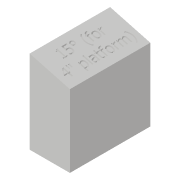
# Autodesk Inventor part: 15DegreeStand
Saved by Autodesk Inventor 2018 (Build 220112000, 112)
## iProperties
Created: 2018-12-13
Part Number: 15DegreeStand
Material: Generic
Document SubType Name: Modeling
Designer: ball
Density: 1 g/cm^3
Appearance: Default
Author: ball
Autodesk Inventor part; units mm, degrees
ref_plane "YZ Plane" through (0, 0, 0) normal (1, 0, 0) x (0, 1, 0)
ref_plane "XZ Plane" through (0, 0, 0) normal (0, 1, 0) x (-1, 0, 0)
ref_plane "XY Plane" through (0, 0, 0) normal (0, 0, 1) x (1, 0, 0)
sketch "Sketch1" plane through (0, 0, 0) normal (0, 1, 0) x (-1, 0, 0)
  line L0 (0, 0) -> (12.7, 0)
  line L1 (12.7, 0) -> (12.7, -25.4)
  line L2 (12.7, -25.4) -> (0, -25.4)
  line L3 (0, -25.4) -> (0, 0)
  dimension "d0" = 12.7
  dimension "d1" = 25.4
  constraints: 8 end point, 2 parallel, 1 horizontal, 1 perpendicular
  measures "d0" distance of L1.end L2.end
  measures "d1" distance of L0.end L1.end
extrude "Extrusion1" add sketch "Sketch1" along normal blind 26.289
sketch "Sketch2" plane through (-12.7, 0, 0) normal (0, 0, 1) x (1, 0, 0)
  line L0 (0, 0) -> (0, 26.289) projected
  line L1 (0, 26.289) -> (12.7, 26.289) projected
  line L2 (0, 26.289) -> (12.7, 26.289)
  line L3 (0, 26.289) -> (12.7, 22.886)
  line L4 (0, 26.289) -> (13.148, 26.289) construction
  line L5 (12.7, 0) -> (12.7, 26.289) projected
  line L6 (12.7, 22.886) -> (12.7, 26.289)
  dimension "d4" = 15
  constraints: 8 end point, 1 collinear, 1 equal length, 1 horizontal, 1 perpendicular
  measures "d4" angle of L3 L4
extrude "Extrusion2" cut sketch "Sketch2" against normal blind 26.289
sketch "Sketch3" plane through (-12.7, 26.289, 0) normal (0.258819, 0.9659258, 0) x (0.9659258, -0.258819, 0)
  line L0 (2.3231, -6.9377) -> (2.3231, 32.6962) construction
  line L1 (2.3231, 32.6962) -> (11.3899, 32.6962) construction
  line L2 (11.3899, 32.6962) -> (11.3899, -6.9377) construction
  line L3 (11.3899, -6.9377) -> (2.3231, -6.9377) construction
  line L4 (5.5267, 6.8821) -> (5.5267, 5.3951)
  line L5 (5.5267, 5.3951) -> (5.2155, 5.3951)
  line L6 (5.2155, 5.3951) -> (5.2155, 5.9484)
  line L7 (5.2155, 5.9484) -> (3.1727, 5.9484)
  line L8 (3.1727, 5.9484) -> (3.1727, 5.3951)
  line L9 (3.1727, 5.3951) -> (2.8936, 5.3951)
  spline S0 degree 2 poles (2.8936, 5.3951) (2.8936, 5.7088) (2.7158, 6.0052) (2.4688, 6.025) knots 0 0 0 1 2 2 2
  line L10 (2.4688, 6.025) -> (2.4688, 6.3411)
  line L11 (2.4688, 6.3411) -> (5.2155, 6.3411)
  line L12 (5.2155, 6.3411) -> (5.2155, 6.8821)
  line L13 (5.2155, 6.8821) -> (5.5267, 6.8821)
  spline S1 degree 2 poles (4.5584, 9.2903) (4.7783, 9.2903) (5.1537, 9.1495) (5.292, 9.0211) knots 0 0 0 1 2 2 2
  spline S2 degree 2 poles (5.292, 9.0211) (5.4303, 8.8927) (5.5909, 8.5098) (5.5909, 8.2727) knots 0 0 0 1 2 2 2
  spline S3 degree 2 poles (5.5909, 8.2727) (5.5909, 8.0553) (5.4946, 7.6305) (5.418, 7.4749) knots 0 0 0 1 2 2 2
  line L14 (5.418, 7.4749) -> (4.9857, 7.4749)
  line L15 (4.9857, 7.4749) -> (4.9857, 7.5045)
  spline S4 degree 2 poles (4.9857, 7.5045) (5.0203, 7.5514) (5.1092, 7.7268) (5.1488, 7.833) knots 0 0 0 1 2 2 2
  spline S5 degree 2 poles (5.1488, 7.833) (5.1907, 7.9541) (5.2377, 8.1541) (5.2377, 8.2801) knots 0 0 0 1 2 2 2
  spline S6 degree 2 poles (5.2377, 8.2801) (5.2377, 8.4036) (5.1488, 8.6358) (5.0524, 8.7198) knots 0 0 0 1 2 2 2
  spline S7 degree 2 poles (5.0524, 8.7198) (4.961, 8.7963) (4.719, 8.8754) (4.556, 8.8754) knots 0 0 0 1 2 2 2
  spline S8 degree 2 poles (4.556, 8.8754) (4.3929, 8.8754) (4.1855, 8.7865) (4.1163, 8.7025) knots 0 0 0 1 2 2 2
  spline S9 degree 2 poles (4.1163, 8.7025) (4.0397, 8.616) (3.9755, 8.3591) (3.9755, 8.2035) knots 0 0 0 1 2 2 2
  spline S10 degree 2 poles (3.9755, 8.2035) (3.9755, 8.0356) (4.0274, 7.7021) (4.0496, 7.6008) knots 0 0 0 1 2 2 2
  line L16 (4.0496, 7.6008) -> (2.4787, 7.6008)
  line L17 (2.4787, 7.6008) -> (2.4787, 9.273)
  line L18 (2.4787, 9.273) -> (2.8368, 9.273)
  line L19 (2.8368, 9.273) -> (2.8368, 7.9936)
  line L20 (2.8368, 7.9936) -> (3.6495, 7.9936)
  spline S11 degree 2 poles (3.6495, 7.9936) (3.6396, 8.0677) (3.6322, 8.2109) (3.6322, 8.2702) knots 0 0 0 1 2 2 2
  spline S12 degree 2 poles (3.6322, 8.2702) (3.6322, 8.5049) (3.7087, 8.8284) (3.8224, 8.9766) knots 0 0 0 1 2 2 2
  spline S13 degree 2 poles (3.8224, 8.9766) (3.936, 9.1273) (4.2818, 9.2903) (4.5584, 9.2903) knots 0 0 0 1 2 2 2
  spline S14 degree 2 poles (3.2049, 11.2738) (3.5334, 11.2738) (3.9829, 10.8242) (3.9829, 10.4957) knots 0 0 0 1 2 2 2
  spline S15 degree 2 poles (3.9829, 10.4957) (3.9829, 10.1697) (3.5358, 9.7152) (3.2049, 9.7152) knots 0 0 0 1 2 2 2
  spline S16 degree 2 poles (3.2049, 9.7152) (2.8763, 9.7152) (2.4268, 10.1647) (2.4268, 10.4957) knots 0 0 0 1 2 2 2
  spline S17 degree 2 poles (2.4268, 10.4957) (2.4268, 10.8242) (2.8763, 11.2738) (3.2049, 11.2738) knots 0 0 0 1 2 2 2
  spline S18 degree 2 poles (3.2049, 10.9527) (3.0073, 10.9527) (2.738, 10.6908) (2.738, 10.4957) knots 0 0 0 1 2 2 2
  spline S19 degree 2 poles (2.738, 10.4957) (2.738, 10.2981) (3.0073, 10.0363) (3.2049, 10.0363) knots 0 0 0 1 2 2 2
  spline S20 degree 2 poles (3.2049, 10.0363) (3.4049, 10.0363) (3.6717, 10.303) (3.6717, 10.4957) knots 0 0 0 1 2 2 2
  spline S21 degree 2 poles (3.6717, 10.4957) (3.6717, 10.6908) (3.4, 10.9527) (3.2049, 10.9527) knots 0 0 0 1 2 2 2
  line L21 (6.3689, 14.2427) -> (6.3689, 13.7734)
  spline S22 degree 2 poles (6.3689, 13.7734) (5.9466, 13.4177) (5.0006, 13.0102) (4.3559, 13.0102) knots 0 0 0 1 2 2 2
  spline S23 degree 2 poles (4.3559, 13.0102) (3.726, 13.0102) (2.7652, 13.4128) (2.3428, 13.7734) knots 0 0 0 1 2 2 2
  line L22 (2.3428, 13.7734) -> (2.3428, 14.2427)
  line L23 (2.3428, 14.2427) -> (2.3626, 14.2427)
  spline S24 degree 2 poles (2.3626, 14.2427) (2.5133, 14.0772) (2.9035, 13.7759) (3.1629, 13.6474) knots 0 0 0 1 2 2 2
  spline S25 degree 2 poles (3.1629, 13.6474) (3.4148, 13.5239) (4.02, 13.3708) (4.3559, 13.3708) knots 0 0 0 1 2 2 2
  spline S26 degree 2 poles (4.3559, 13.3708) (4.7066, 13.3708) (5.2871, 13.519) (5.5489, 13.6474) knots 0 0 0 1 2 2 2
  spline S27 degree 2 poles (5.5489, 13.6474) (5.8008, 13.7709) (6.2084, 14.0846) (6.3492, 14.2427) knots 0 0 0 1 2 2 2
  line L24 (6.3492, 14.2427) -> (6.3689, 14.2427)
  line L25 (2.7133, 15.8779) -> (2.7133, 15.8581)
  spline S28 degree 2 poles (2.7133, 15.8581) (2.6936, 15.8062) (2.659, 15.6136) (2.659, 15.537) knots 0 0 0 1 2 2 2
  spline S29 degree 2 poles (2.659, 15.537) (2.659, 15.2949) (2.8763, 15.0875) (3.1629, 15.0875) knots 0 0 0 1 2 2 2
  line L26 (3.1629, 15.0875) -> (3.2394, 15.0875)
  line L27 (3.2394, 15.0875) -> (3.2394, 15.7247)
  line L28 (3.2394, 15.7247) -> (3.5581, 15.7247)
  line L29 (3.5581, 15.7247) -> (3.5581, 15.0998)
  line L30 (3.5581, 15.0998) -> (5.5267, 15.0998)
  line L31 (5.5267, 15.0998) -> (5.5267, 14.7145)
  line L32 (5.5267, 14.7145) -> (3.5581, 14.7145)
  line L33 (3.5581, 14.7145) -> (3.5581, 14.4551)
  line L34 (3.5581, 14.4551) -> (3.2394, 14.4551)
  line L35 (3.2394, 14.4551) -> (3.2394, 14.7145)
  line L36 (3.2394, 14.7145) -> (3.1629, 14.7145)
  spline S30 degree 2 poles (3.1629, 14.7145) (2.7528, 14.7145) (2.3231, 15.1122) (2.3231, 15.4827) knots 0 0 0 1 2 2 2
  spline S31 degree 2 poles (2.3231, 15.4827) (2.3231, 15.5889) (2.3453, 15.7939) (2.3601, 15.8779) knots 0 0 0 1 2 2 2
  line L37 (2.3601, 15.8779) -> (2.7133, 15.8779)
  spline S32 degree 2 poles (4.3831, 17.8885) (4.961, 17.8885) (5.5909, 17.3327) (5.5909, 16.8683) knots 0 0 0 1 2 2 2
  spline S33 degree 2 poles (5.5909, 16.8683) (5.5909, 16.3916) (4.9413, 15.8458) (4.3831, 15.8458) knots 0 0 0 1 2 2 2
  spline S34 degree 2 poles (4.3831, 15.8458) (3.81, 15.8458) (3.1752, 16.4089) (3.1752, 16.8683) knots 0 0 0 1 2 2 2
  spline S35 degree 2 poles (3.1752, 16.8683) (3.1752, 17.3327) (3.8075, 17.8885) (4.3831, 17.8885) knots 0 0 0 1 2 2 2
  spline S36 degree 2 poles (4.3831, 17.4908) (3.9385, 17.4908) (3.5062, 17.1672) (3.5062, 16.8683) knots 0 0 0 1 2 2 2
  spline S37 degree 2 poles (3.5062, 16.8683) (3.5062, 16.5695) (3.9385, 16.2434) (4.3831, 16.2434) knots 0 0 0 1 2 2 2
  spline S38 degree 2 poles (4.3831, 16.2434) (4.8153, 16.2434) (5.2599, 16.5695) (5.2599, 16.8683) knots 0 0 0 1 2 2 2
  spline S39 degree 2 poles (5.2599, 16.8683) (5.2599, 17.1647) (4.8227, 17.4908) (4.3831, 17.4908) knots 0 0 0 1 2 2 2
  line L38 (3.6519, 19.4964) -> (3.6519, 19.4767)
  spline S40 degree 2 poles (3.6519, 19.4767) (3.6396, 19.4322) (3.6346, 19.3359) (3.6346, 19.2692) knots 0 0 0 1 2 2 2
  spline S41 degree 2 poles (3.6346, 19.2692) (3.6346, 19.1136) (3.7705, 18.8073) (3.9039, 18.669) knots 0 0 0 1 2 2 2
  line L39 (3.9039, 18.669) -> (5.5267, 18.669)
  line L40 (5.5267, 18.669) -> (5.5267, 18.2837)
  line L41 (5.5267, 18.2837) -> (3.2394, 18.2837)
  line L42 (3.2394, 18.2837) -> (3.2394, 18.669)
  line L43 (3.2394, 18.669) -> (3.5803, 18.669)
  spline S42 degree 2 poles (3.5803, 18.669) (3.3926, 18.8789) (3.2394, 19.1926) (3.2394, 19.3408) knots 0 0 0 1 2 2 2
  spline S43 degree 2 poles (3.2394, 19.3408) (3.2394, 19.4001) (3.2444, 19.4594) (3.2518, 19.4964) knots 0 0 0 1 2 2 2
  line L44 (3.2518, 19.4964) -> (3.6519, 19.4964)
  line L45 (9.4978, 3.8612) -> (9.4978, 3.4981)
  line L46 (9.4978, 3.4981) -> (10.5451, 3.4981)
  line L47 (10.5451, 3.4981) -> (10.5451, 3.1054)
  line L48 (10.5451, 3.1054) -> (9.4978, 3.1054)
  line L49 (9.4978, 3.1054) -> (9.4978, 1.7593)
  line L50 (9.4978, 1.7593) -> (9.0681, 1.7593)
  line L51 (9.0681, 1.7593) -> (7.4971, 3.1227)
  line L52 (7.4971, 3.1227) -> (7.4971, 3.4981)
  line L53 (7.4971, 3.4981) -> (9.1693, 3.4981)
  line L54 (9.1693, 3.4981) -> (9.1693, 3.8612)
  line L55 (9.1693, 3.8612) -> (9.4978, 3.8612)
  line L56 (9.1693, 3.1054) -> (7.9788, 3.1054)
  line L57 (7.9788, 3.1054) -> (9.1693, 2.0804)
  line L58 (9.1693, 2.0804) -> (9.1693, 3.1054)
  line L59 (7.3613, 4.6442) -> (8.5469, 4.5553)
  line L60 (8.5469, 4.5553) -> (8.5469, 4.2861)
  line L61 (8.5469, 4.2861) -> (7.3613, 4.1972)
  line L62 (7.3613, 4.1972) -> (7.3613, 4.6442)
  line L63 (7.3613, 5.4149) -> (8.5469, 5.326)
  line L64 (8.5469, 5.326) -> (8.5469, 5.0567)
  line L65 (8.5469, 5.0567) -> (7.3613, 4.9678)
  line L66 (7.3613, 4.9678) -> (7.3613, 5.4149)
  spline S44 degree 2 poles (9.3398, 9.152) (9.9128, 9.152) (10.5896, 8.6061) (10.5896, 8.1887) knots 0 0 0 1 2 2 2
  spline S45 degree 2 poles (10.5896, 8.1887) (10.5896, 8.0183) (10.5105, 7.7565) (10.429, 7.6206) knots 0 0 0 1 2 2 2
  line L67 (10.429, 7.6206) -> (11.3874, 7.6206)
  line L68 (11.3874, 7.6206) -> (11.3874, 7.2353)
  line L69 (11.3874, 7.2353) -> (8.2579, 7.2353)
  line L70 (8.2579, 7.2353) -> (8.2579, 7.6206)
  line L71 (8.2579, 7.6206) -> (8.4975, 7.6206)
  spline S46 degree 2 poles (8.4975, 7.6206) (8.3666, 7.7639) (8.1937, 8.1146) (8.1937, 8.3196) knots 0 0 0 1 2 2 2
  spline S47 degree 2 poles (8.1937, 8.3196) (8.1937, 8.7124) (8.8161, 9.152) (9.3398, 9.152) knots 0 0 0 1 2 2 2
  spline S48 degree 2 poles (9.3842, 8.7543) (8.9915, 8.7543) (8.5592, 8.5049) (8.5592, 8.2258) knots 0 0 0 1 2 2 2
  spline S49 degree 2 poles (8.5592, 8.2258) (8.5592, 8.0627) (8.705, 7.7565) (8.8186, 7.6206) knots 0 0 0 1 2 2 2
  line L72 (8.8186, 7.6206) -> (10.1178, 7.6206)
  spline S50 degree 2 poles (10.1178, 7.6206) (10.1894, 7.7713) (10.2438, 7.9862) (10.2438, 8.1245) knots 0 0 0 1 2 2 2
  spline S51 degree 2 poles (10.2438, 8.1245) (10.2438, 8.4234) (9.8041, 8.7543) (9.3842, 8.7543) knots 0 0 0 1 2 2 2
  line L73 (10.5451, 9.9449) -> (10.5451, 9.5596)
  line L74 (10.5451, 9.5596) -> (7.3613, 9.5596)
  line L75 (7.3613, 9.5596) -> (7.3613, 9.9449)
  line L76 (7.3613, 9.9449) -> (10.5451, 9.9449)
  spline S52 degree 2 poles (10.3031, 11.7851) (10.3376, 11.7381) (10.4611, 11.58) (10.4982, 11.5059) knots 0 0 0 1 2 2 2
  spline S53 degree 2 poles (10.4982, 11.5059) (10.5525, 11.4047) (10.6093, 11.2145) (10.6093, 11.0416) knots 0 0 0 1 2 2 2
  spline S54 degree 2 poles (10.6093, 11.0416) (10.6093, 10.9008) (10.5031, 10.6464) (10.4068, 10.55) knots 0 0 0 1 2 2 2
  spline S55 degree 2 poles (10.4068, 10.55) (10.3129, 10.4587) (10.0363, 10.3475) (9.8832, 10.3475) knots 0 0 0 1 2 2 2
  spline S56 degree 2 poles (9.8832, 10.3475) (9.646, 10.3475) (9.3101, 10.5476) (9.2138, 10.7649) knots 0 0 0 1 2 2 2
  spline S57 degree 2 poles (9.2138, 10.7649) (9.1249, 10.9576) (9.0582, 11.4812) (9.0409, 11.7851) knots 0 0 0 1 2 2 2
  line L77 (9.0409, 11.7851) -> (8.9668, 11.7851)
  spline S58 degree 2 poles (8.9668, 11.7851) (8.8334, 11.7851) (8.6679, 11.7035) (8.621, 11.6294) knots 0 0 0 1 2 2 2
  spline S59 degree 2 poles (8.621, 11.6294) (8.5741, 11.5553) (8.5444, 11.3429) (8.5444, 11.2293) knots 0 0 0 1 2 2 2
  spline S60 degree 2 poles (8.5444, 11.2293) (8.5444, 11.0959) (8.6235, 10.7353) (8.7, 10.555) knots 0 0 0 1 2 2 2
  line L78 (8.7, 10.555) -> (8.7, 10.5328)
  line L79 (8.7, 10.5328) -> (8.3073, 10.5328)
  spline S61 degree 2 poles (8.3073, 10.5328) (8.2776, 10.639) (8.2035, 11.0366) (8.2035, 11.2318) knots 0 0 0 1 2 2 2
  spline S62 degree 2 poles (8.2035, 11.2318) (8.2035, 11.4689) (8.2776, 11.7925) (8.374, 11.9209) knots 0 0 0 1 2 2 2
  spline S63 degree 2 poles (8.374, 11.9209) (8.4678, 12.0469) (8.7667, 12.1704) (8.9816, 12.1704) knots 0 0 0 1 2 2 2
  line L80 (8.9816, 12.1704) -> (10.5451, 12.1704)
  line L81 (10.5451, 12.1704) -> (10.5451, 11.7851)
  line L82 (10.5451, 11.7851) -> (10.3031, 11.7851)
  line L83 (9.982, 11.7851) -> (9.3472, 11.7851)
  spline S64 degree 2 poles (9.3472, 11.7851) (9.3595, 11.6467) (9.4015, 11.2293) (9.441, 11.0984) knots 0 0 0 1 2 2 2
  spline S65 degree 2 poles (9.441, 11.0984) (9.488, 10.9452) (9.6831, 10.7452) (9.856, 10.7452) knots 0 0 0 1 2 2 2
  spline S66 degree 2 poles (9.856, 10.7452) (10.0536, 10.7452) (10.2537, 10.9675) (10.2537, 11.1799) knots 0 0 0 1 2 2 2
  spline S67 degree 2 poles (10.2537, 11.1799) (10.2537, 11.3602) (10.0981, 11.6566) (9.982, 11.7851) knots 0 0 0 1 2 2 2
  spline S68 degree 2 poles (10.5896, 13.4029) (10.5896, 13.0892) (10.2314, 12.736) (9.8436, 12.736) knots 0 0 0 1 2 2 2
  line L84 (9.8436, 12.736) -> (8.5765, 12.736)
  line L85 (8.5765, 12.736) -> (8.5765, 12.4767)
  line L86 (8.5765, 12.4767) -> (8.2579, 12.4767)
  line L87 (8.2579, 12.4767) -> (8.2579, 12.736)
  line L88 (8.2579, 12.736) -> (7.6009, 12.736)
  line L89 (7.6009, 12.736) -> (7.6009, 13.1213)
  line L90 (7.6009, 13.1213) -> (8.2579, 13.1213)
  line L91 (8.2579, 13.1213) -> (8.2579, 13.8302)
  line L92 (8.2579, 13.8302) -> (8.5765, 13.8302)
  line L93 (8.5765, 13.8302) -> (8.5765, 13.1213)
  line L94 (8.5765, 13.1213) -> (9.6658, 13.1213)
  spline S69 degree 2 poles (9.6658, 13.1213) (9.8387, 13.1213) (10.0289, 13.1337) (10.1104, 13.1757) knots 0 0 0 1 2 2 2
  spline S70 degree 2 poles (10.1104, 13.1757) (10.182, 13.2103) (10.2537, 13.3659) (10.2537, 13.4992) knots 0 0 0 1 2 2 2
  spline S71 degree 2 poles (10.2537, 13.4992) (10.2537, 13.5931) (10.1969, 13.7685) (10.1796, 13.808) knots 0 0 0 1 2 2 2
  line L95 (10.1796, 13.808) -> (10.1796, 13.8302)
  line L96 (10.1796, 13.8302) -> (10.5254, 13.8302)
  spline S72 degree 2 poles (10.5254, 13.8302) (10.555, 13.7215) (10.5896, 13.4992) (10.5896, 13.4029) knots 0 0 0 1 2 2 2
  line L97 (7.7318, 15.3172) -> (7.7318, 15.2974)
  spline S73 degree 2 poles (7.7318, 15.2974) (7.712, 15.2455) (7.6774, 15.0529) (7.6774, 14.9763) knots 0 0 0 1 2 2 2
  spline S74 degree 2 poles (7.6774, 14.9763) (7.6774, 14.7343) (7.8948, 14.5268) (8.1813, 14.5268) knots 0 0 0 1 2 2 2
  line L98 (8.1813, 14.5268) -> (8.2579, 14.5268)
  line L99 (8.2579, 14.5268) -> (8.2579, 15.164)
  line L100 (8.2579, 15.164) -> (8.5765, 15.164)
  line L101 (8.5765, 15.164) -> (8.5765, 14.5391)
  line L102 (8.5765, 14.5391) -> (10.5451, 14.5391)
  line L103 (10.5451, 14.5391) -> (10.5451, 14.1538)
  line L104 (10.5451, 14.1538) -> (8.5765, 14.1538)
  line L105 (8.5765, 14.1538) -> (8.5765, 13.8944)
  line L106 (8.5765, 13.8944) -> (8.2579, 13.8944)
  line L107 (8.2579, 13.8944) -> (8.2579, 14.1538)
  line L108 (8.2579, 14.1538) -> (8.1813, 14.1538)
  spline S75 degree 2 poles (8.1813, 14.1538) (7.7713, 14.1538) (7.3415, 14.5515) (7.3415, 14.922) knots 0 0 0 1 2 2 2
  spline S76 degree 2 poles (7.3415, 14.922) (7.3415, 15.0282) (7.3637, 15.2332) (7.3786, 15.3172) knots 0 0 0 1 2 2 2
  line L109 (7.3786, 15.3172) -> (7.7318, 15.3172)
  spline S77 degree 2 poles (9.4015, 17.3278) (9.9795, 17.3278) (10.6093, 16.772) (10.6093, 16.3077) knots 0 0 0 1 2 2 2
  spline S78 degree 2 poles (10.6093, 16.3077) (10.6093, 15.8309) (9.9597, 15.2851) (9.4015, 15.2851) knots 0 0 0 1 2 2 2
  spline S79 degree 2 poles (9.4015, 15.2851) (8.8285, 15.2851) (8.1937, 15.8482) (8.1937, 16.3077) knots 0 0 0 1 2 2 2
  spline S80 degree 2 poles (8.1937, 16.3077) (8.1937, 16.772) (8.826, 17.3278) (9.4015, 17.3278) knots 0 0 0 1 2 2 2
  spline S81 degree 2 poles (9.4015, 16.9301) (8.9569, 16.9301) (8.5247, 16.6065) (8.5247, 16.3077) knots 0 0 0 1 2 2 2
  spline S82 degree 2 poles (8.5247, 16.3077) (8.5247, 16.0088) (8.9569, 15.6827) (9.4015, 15.6827) knots 0 0 0 1 2 2 2
  spline S83 degree 2 poles (9.4015, 15.6827) (9.8338, 15.6827) (10.2784, 16.0088) (10.2784, 16.3077) knots 0 0 0 1 2 2 2
  spline S84 degree 2 poles (10.2784, 16.3077) (10.2784, 16.6041) (9.8412, 16.9301) (9.4015, 16.9301) knots 0 0 0 1 2 2 2
  line L110 (8.6704, 18.9357) -> (8.6704, 18.916)
  spline S85 degree 2 poles (8.6704, 18.916) (8.658, 18.8715) (8.6531, 18.7752) (8.6531, 18.7085) knots 0 0 0 1 2 2 2
  spline S86 degree 2 poles (8.6531, 18.7085) (8.6531, 18.5529) (8.7889, 18.2466) (8.9223, 18.1083) knots 0 0 0 1 2 2 2
  line L111 (8.9223, 18.1083) -> (10.5451, 18.1083)
  line L112 (10.5451, 18.1083) -> (10.5451, 17.723)
  line L113 (10.5451, 17.723) -> (8.2579, 17.723)
  line L114 (8.2579, 17.723) -> (8.2579, 18.1083)
  line L115 (8.2579, 18.1083) -> (8.5988, 18.1083)
  spline S87 degree 2 poles (8.5988, 18.1083) (8.411, 18.3182) (8.2579, 18.6319) (8.2579, 18.7801) knots 0 0 0 1 2 2 2
  spline S88 degree 2 poles (8.2579, 18.7801) (8.2579, 18.8394) (8.2628, 18.8987) (8.2702, 18.9357) knots 0 0 0 1 2 2 2
  line L116 (8.2702, 18.9357) -> (8.6704, 18.9357)
  line L117 (10.5451, 21.8281) -> (9.2212, 21.8281)
  spline S89 degree 2 poles (9.2212, 21.8281) (9.0631, 21.8281) (8.7939, 21.8034) (8.7198, 21.7639) knots 0 0 0 1 2 2 2
  spline S90 degree 2 poles (8.7198, 21.7639) (8.6383, 21.7244) (8.5592, 21.5737) (8.5592, 21.4428) knots 0 0 0 1 2 2 2
  spline S91 degree 2 poles (8.5592, 21.4428) (8.5592, 21.3243) (8.705, 21.0526) (8.8433, 20.9093) knots 0 0 0 1 2 2 2
  spline S92 degree 2 poles (8.8433, 20.9093) (8.8779, 20.9118) (8.9742, 20.9167) (9.0384, 20.9167) knots 0 0 0 1 2 2 2
  line L118 (9.0384, 20.9167) -> (10.5451, 20.9167)
  line L119 (10.5451, 20.9167) -> (10.5451, 20.5314)
  line L120 (10.5451, 20.5314) -> (9.2212, 20.5314)
  spline S93 degree 2 poles (9.2212, 20.5314) (9.0631, 20.5314) (8.7939, 20.5067) (8.7198, 20.4672) knots 0 0 0 1 2 2 2
  spline S94 degree 2 poles (8.7198, 20.4672) (8.6383, 20.4276) (8.5592, 20.277) (8.5592, 20.1461) knots 0 0 0 1 2 2 2
  spline S95 degree 2 poles (8.5592, 20.1461) (8.5592, 20.0226) (8.7148, 19.7484) (8.8359, 19.6199) knots 0 0 0 1 2 2 2
  line L121 (8.8359, 19.6199) -> (10.5451, 19.6199)
  line L122 (10.5451, 19.6199) -> (10.5451, 19.2346)
  line L123 (10.5451, 19.2346) -> (8.2579, 19.2346)
  line L124 (8.2579, 19.2346) -> (8.2579, 19.6199)
  line L125 (8.2579, 19.6199) -> (8.5098, 19.6199)
  spline S96 degree 2 poles (8.5098, 19.6199) (8.3592, 19.7706) (8.1937, 20.067) (8.1937, 20.2449) knots 0 0 0 1 2 2 2
  spline S97 degree 2 poles (8.1937, 20.2449) (8.1937, 20.4474) (8.3789, 20.7611) (8.5889, 20.8426) knots 0 0 0 1 2 2 2
  spline S98 degree 2 poles (8.5889, 20.8426) (8.3937, 21.018) (8.1937, 21.349) (8.1937, 21.5416) knots 0 0 0 1 2 2 2
  spline S99 degree 2 poles (8.1937, 21.5416) (8.1937, 21.6898) (8.2851, 21.9319) (8.3888, 22.0208) knots 0 0 0 1 2 2 2
  spline S100 degree 2 poles (8.3888, 22.0208) (8.4925, 22.1122) (8.8038, 22.2135) (9.0384, 22.2135) knots 0 0 0 1 2 2 2
  line L126 (9.0384, 22.2135) -> (10.5451, 22.2135)
  line L127 (10.5451, 22.2135) -> (10.5451, 21.8281)
  spline S101 degree 2 poles (9.3743, 23.861) (10.0067, 23.861) (10.965, 23.4559) (11.3874, 23.0977) knots 0 0 0 1 2 2 2
  line L128 (11.3874, 23.0977) -> (11.3874, 22.6284)
  line L129 (11.3874, 22.6284) -> (11.3676, 22.6284)
  spline S102 degree 2 poles (11.3676, 22.6284) (11.2268, 22.7865) (10.8144, 23.1051) (10.5674, 23.2237) knots 0 0 0 1 2 2 2
  spline S103 degree 2 poles (10.5674, 23.2237) (10.3031, 23.3521) (9.7152, 23.5003) (9.3743, 23.5003) knots 0 0 0 1 2 2 2
  spline S104 degree 2 poles (9.3743, 23.5003) (9.0359, 23.5003) (8.4357, 23.3497) (8.1813, 23.2237) knots 0 0 0 1 2 2 2
  spline S105 degree 2 poles (8.1813, 23.2237) (7.9269, 23.1002) (7.5218, 22.784) (7.381, 22.6284) knots 0 0 0 1 2 2 2
  line L130 (7.381, 22.6284) -> (7.3613, 22.6284)
  line L131 (7.3613, 22.6284) -> (7.3613, 23.0977)
  spline S106 degree 2 poles (7.3613, 23.0977) (7.7836, 23.4534) (8.7371, 23.861) (9.3743, 23.861) knots 0 0 0 1 2 2 2
  point P0 (19.0714, 0)
  constraints: 2 other
emboss "Emboss1" sketch "Sketch3" operation cut depth 1.016 direction (-0.258819, -0.9659258, 0)
body "Solid1"
